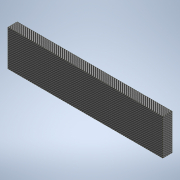
# Autodesk Inventor part: 007
Saved by Autodesk Inventor 2022.2 (Build 262287000, 287)
## iProperties
Manager: Angie Guevara
Company: ITM
Created: 2021-11-08
Part Number: 007
Material: GFRC
Document SubType Name: Modeling
Designer: Samuel Gómez
Density: 1.7 g/cm^3
Appearance: Carbon Fiber 1
Checked By: Angie Guevara
Engr Approved By: Angie Guevara
Engineer: Angie Guevara
Author: Samuel Gómez
Title: Placa2
Autodesk Inventor part; units mm, degrees
ref_plane "YZ Plane" through (0, 0, 0) normal (1, 0, 0) x (0, 1, 0)
ref_plane "XZ Plane" through (0, 0, 0) normal (0, 1, 0) x (-1, 0, 0)
ref_plane "XY Plane" through (0, 0, 0) normal (0, 0, 1) x (1, 0, 0)
sketch "Boceto1" plane through (0, 0, 0) normal (0, 0, 1) x (1, 0, 0)
  line L0 (0, 0) -> (300, 0)
  line L1 (300, 0) -> (300, -70)
  line L2 (300, -70) -> (0, -70)
  line L3 (0, -70) -> (0, 0)
  dimension "d0" = 300
  dimension "d1" = 70
  constraints: 8 end point, 2 parallel, 1 horizontal, 1 perpendicular
  measures "d0" distance of L0.start L0.end
  measures "d1" distance of L2.end L0.start
extrude "Extrusión1" add sketch "Boceto1" along normal blind 18
